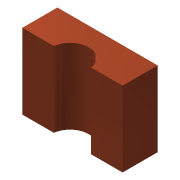
# Autodesk Inventor part: 17-0028-0110
Saved by Autodesk Inventor 2016 SP2 (Build 200236200, 236)
## iProperties
Category: IOP
Company: Universiteit van Amsterdam
Created: 2017-12-29
Part Number: 17-0028-0110
Material: Copper
Document SubType Name: Modeling
Designer: Daan Giesen
Density: 8.94 g/cm^3
Appearance: Copper - Satin
Project: Digital PID Loop
Cost Center: 17-0028
User Status: Work in Progress
Authority: Reichsöllner, Lukas
Author: Daan Giesen
Title: Digital PID Loop
Revision Number: A
Autodesk Inventor part; units mm, degrees
ref_plane "YZ Plane" through (0, 0, 0) normal (1, 0, 0) x (0, 1, 0)
ref_plane "XZ Plane" through (0, 0, 0) normal (0, 1, 0) x (-1, 0, 0)
ref_plane "XY Plane" through (0, 0, 0) normal (0, 0, 1) x (1, 0, 0)
sketch "Sketch1" plane through (0, 0, 0) normal (0, 0, 1) x (1, 0, 0)
  line L0 (0, 19.5) -> (0, -12) construction
  line L1 (-28, 0) -> (28, 0) construction
  line L2 (20, 15) -> (-20, 15)
  line L3 (-20, 15) -> (-20, 1)
  line L4 (20, 1) -> (20, 15)
  line L5 (20, 15) -> (-20, 1) construction
  line L6 (-20, 15) -> (20, 1) construction
  circle A0 centre (0, 0) radius 7.5
  line L7 (-20, 1) -> (-7.433, 1)
  line L8 (7.433, 1) -> (20, 1)
  point P0 (0, 8)
  dimension "d4" = 40
  dimension "d5" = 14
  dimension "d6" = 15
  dimension "d8" = 1
  constraints: 14 end point, 3 parallel, 2 midpoint, 2 point on circle, 1 centre point, 1 coincident, 1 horizontal, 1 horizontal alignment, 1 perpendicular, 1 point on line
  measures "d4" distance of L2.start L2.end
  measures "d5" distance of L4.start L2.start
  measures "d6" diameter of A0
  measures "d8" distance from line of point (0, 0) L8
extrude "Extrusion3" add sketch "Sketch1" against normal blind 30 contours L4 L8 A0 L7 L3 L2
sketch "Sketch2" plane through (-20, 15, 0) normal (0, 1, 0) x (1, 0, 0)
  line L0 (32.5, 7.5) -> (7.5, 7.5) construction
  line L1 (7.5, 7.5) -> (7.5, 22.5) construction
  line L2 (7.5, 22.5) -> (32.5, 22.5) construction
  line L3 (32.5, 22.5) -> (32.5, 7.5) construction
  line L4 (32.5, 7.5) -> (7.5, 22.5) construction
  line L5 (7.5, 7.5) -> (32.5, 22.5) construction
  line L6 (40, 0) -> (0, 0) construction
  point P0 (20, 0)
  point P1 (20, 15)
  point P2 (20, 15)
  point P3 (20, 0)
  dimension "d11" = 15
  dimension "d12" = 25
  dimension "d13" = 15
  constraints: 12 end point, 4 coincident, 4 midpoint, 2 parallel, 1 horizontal, 1 perpendicular, 1 vertical alignment
  measures "d11" distance of L2.end L0.start
  measures "d12" distance of L1.end L2.end
  measures "d13" distance of point (20, 15) point (20, 0)
sketch "Sketch3" plane through (-20, 15, 0) normal (0, 1, 0) x (1, 0, 0)
  point P0 (7.5, 22.5)
  point P1 (32.5, 22.5)
  point P2 (32.5, 7.5)
  point P3 (7.5, 7.5)
hole "Hole1" at (-12.5, 15, -22.5) at (12.5, 15, -22.5) at (12.5, 15, -7.5) at (-12.5, 15, -7.5) direction (0, -1, 0) diameter 5.5 depth 14 counterbore diameter 10 counterbore depth 5.7
body "Solid3"
